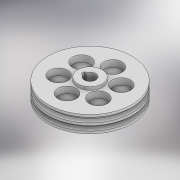
# Autodesk Inventor part: 1
Saved by Autodesk Inventor 2020 (Build 240168000, 168)
## iProperties
Created: 2021-03-24
Part Number: 1
Material: 常规
Document SubType Name: Modeling
Designer: Luorily
Density: 1 g/cm^3
Appearance: 默认
Author: Luorily
Autodesk Inventor part; units mm, degrees
ref_plane "YZ Plane" through (0, 0, 0) normal (1, 0, 0) x (0, 1, 0)
ref_plane "XZ Plane" through (0, 0, 0) normal (0, 1, 0) x (-1, 0, 0)
ref_plane "XY Plane" through (0, 0, 0) normal (0, 0, 1) x (1, 0, 0)
sketch "草图1" plane through (0, 0, 0) normal (0, 0, 1) x (1, 0, 0)
  line L0 (0, 0) -> (0, 30)
  line L1 (0, 30) -> (-16, 30)
  line L2 (-16, 30) -> (-16, 26)
  line L3 (-16, 26) -> (-55, 26)
  line L4 (-54.8586, 22.861) -> (-50.0487, 20.9752)
  line L5 (-50.0487, 20.9752) -> (-50.0487, 17.9752)
  line L6 (-50.0487, 17.9752) -> (-55, 16.5)
  line L7 (0, 0) -> (-16, 0)
  line L8 (-16, 0) -> (-16, 4)
  line L9 (-16, 4) -> (-55, 4)
  line L10 (-55, 13.5) -> (-50.0487, 12.0248)
  line L11 (-50.0487, 12.0248) -> (-50.0487, 9.0248)
  line L12 (-50.0487, 9.0248) -> (-54.8586, 7.139)
  line L13 (-55, 16.5) -> (-55, 13.5)
  line L14 (-54.8586, 4) -> (-54.8586, 7.139)
  line L15 (-54.8586, 26) -> (-54.8586, 22.861)
  point P0 (-54.9901, 12.2219)
  dimension "d0" = 30
  dimension "d1" = 16
  dimension "d2" = 4
  dimension "d3" = 39
  dimension "d4" = 22
  dimension "d5" = 38
  dimension "d7" = 3
  dimension "d8" = 38
  dimension "d9" = 3
  constraints: 32 end point, 4 point on line, 4 vertical, 3 equal length, 3 perpendicular, 1 collinear, 1 parallel
  measures "d0" distance of L0.start L0.end
  measures "d1" distance of L0.end L1.end
  measures "d2" distance of L1.end L2.end
  measures "d3" distance of L2.end L3.end
  measures "d4" distance of L3.end L9.end
  measures "d5" angle of L6 L4
  measures "d7" distance of L4.end L5.end
  measures "d8" angle of L12 L10
  measures "d9" distance of L11.start L12.start
revolve "旋转1" add sketch "草图1" angle 360 about axis through (0, 0, 0) along (0, 1, 0)
sketch "草图2" plane through (0, 26, 0) normal (0, 1, 0) x (1, 0, 0)
  circle A0 centre (0, 0) radius 54.8586 projected
  circle A1 centre (0, 0) radius 16 projected
  circle A2 centre (0, 0) radius 30
  circle A3 centre (0, -30) radius 12
  circle A4 centre (25.9808, -15) radius 12
  circle A5 centre (25.9808, 15) radius 12
  circle A6 centre (0, 30) radius 12
  circle A7 centre (-25.9808, 15) radius 12
  circle A8 centre (-25.9808, -15) radius 12
  dimension "d14" = 24
  dimension "d17" = 360
  constraints: 6 centre point, 1 coincident, 1 vertical alignment, 15 other
  measures "d14" diameter of A3
sketch "草图3" plane through (0, 0, 0) normal (0, -1, 0) x (1, 0, 0)
  circle A0 centre (0, 0) radius 16 projected
  arc A1 (-7.2284, -2) -> (-7.2284, 2) centre (0, 0) ccw
  line L0 (-9.6, 0) -> (-9.6, 2)
  line L1 (-9.6, 2) -> (-9.6, -2)
  line L2 (-9.6, -2) -> (-7.2284, -2)
  line L3 (-9.6, 2) -> (-7.2284, 2)
  dimension "d19" = 15
  dimension "d20" = 9.6
  dimension "d21" = 2
  dimension "d22" = 4
  constraints: 8 end point, 2 point on circle, 1 centre point, 1 coincident, 1 parallel, 1 perpendicular, 1 point on line
  measures "d19" diameter of A1
  measures "d20" distance of A1.centre L0.start
  measures "d21" distance of L0.start L0.end
  measures "d22" distance of L0.end L1.end
extrude "拉伸1" cut sketch "草图3" against normal through all contours L2 L1 L0 L3 A1
extrude "拉伸2" cut sketch "草图2" against normal blind 8.74 contours A5 A2 | A2 A5 | A4 A2 | A2 A4 | A6 A2 | A2 A6 | A3 A2 | A2 A3 | A7 A2 | A2 A7 | A8 A2 | A2 A8
sketch "草图4" plane through (0, 4, 0) normal (0, -1, 0) x (1, 0, 0)
  circle A0 centre (0, 0) radius 16 projected
  circle A1 centre (-25.9808, -15) radius 12 projected
  circle A2 centre (-25.9808, 15) radius 12 projected
  circle A3 centre (0, 30) radius 12 projected
  point P0 (0, 30)
  point P1 (25.9808, 15)
  point P2 (25.9808, -15)
  point P3 (0, -30)
  point P4 (-25.9808, -15)
  dimension "d29" = 360
  constraints: 5 coincident, 11 other
hole "孔1" at (-25.9808, 4, 15) at (0, 4, 30) at (25.9808, 4, 15) at (25.9808, 4, -15) at (0, 4, -30) at (-25.9808, 4, -15) direction (0, 1, 0) diameter 24 depth 8.74
